door_puller_anchor (Autodesk Fusion 360 design; units mm, degrees)
Autodesk Fusion 360 part; units mm, degrees
note: some values were not read from the file. Set by a fixed rule: which sketch regions a step uses.
sketch "Sketch1" plane through (0, 0, 0) normal (0, 0, 1) x (1, 0, 0)
  line L0 (20, -10) -> (-20, -10)
  line L1 (-20, -10) -> (-20, 10)
  line L2 (-20, 10) -> (20, 10)
  line L3 (20, 10) -> (20, -10)
  line L4 (20, -10) -> (-20, 10) construction
  line L5 (-20, -10) -> (20, 10) construction
  line L6 (10, 10) -> (10, -10)
  line L7 (-10, 10) -> (-10, -10) construction
  circle A0 centre (-10, 0) radius 1.7
  circle A1 centre (-10, 0) radius 3
  circle A2 centre (10, 0) radius 1.45
  circle A3 centre (10, 0) radius 3
  line L8 (-20, 3) -> (20, 3)
  line L9 (-20, -3) -> (20, -3)
  circle A4 centre (10, 0) radius 6
  line L10 (13, 5.1962) -> (13, 10)
  line L11 (7, 5.1962) -> (7, 10)
  line L12 (-7, 3) -> (-7, -3)
  line L13 (7, 3) -> (7, -3)
  line L14 (0, 10) -> (0, -10)
  line L15 (-20, 10) -> (-40, 10)
  line L16 (-40, 10) -> (-40, -10)
  line L17 (-40, -10) -> (-20, -10)
  line L18 (-40, 0) -> (-20, 0) construction
  circle A5 centre (-30, 0) radius 1.7
  circle A6 centre (-30, 0) radius 3
  dimension "d1" = 40
  dimension "d2" = 20
  dimension "d3" = 10
  dimension "d4" = 10
  dimension "d5" = 3.4
  dimension "d6" = 6
  dimension "d7" = 12
  dimension "d8" = 6
  dimension "d15" = 2.9
  dimension "d36" = 20
  constraint horizontal L0
  constraint parallel L0 L2
  constraint parallel L1 L3
  constraint coincident L4 origin
  constraint coincident L5 origin
  constraint coincident L2 L6.start
  constraint coincident L0 L6.end
  constraint vertical L6
  constraint coincident L2 L7.start
  constraint coincident L0 L7.end
  constraint vertical L1
  constraint vertical L7
  constraint midpoint L7 A0.centre
  constraint concentric A0 A1
  constraint coincident L6 A2.centre
  constraint concentric A2 A3
  constraint equal A1 A3
  constraint midpoint L6 A2.centre
  constraint coincident L1 L8.start
  constraint coincident L3 L8.end
  constraint horizontal L8
  constraint tangent A3 L8
  constraint coincident L1 L9.start
  constraint coincident L3 L9.end
  constraint horizontal L9
  constraint tangent A3 L9
  constraint concentric A2 A4
  constraint coincident A4 L10.start
  constraint coincident L2 L10.end
  constraint vertical L10
  constraint symmetric L6 L10.start L11.start
  constraint symmetric L6 L10.end L11.end
  constraint coincident L2 L11.end
  constraint coincident L8 L12.start
  constraint coincident L9 L12.end
  constraint vertical L12
  constraint coincident L8 L13.start
  constraint coincident L9 L13.end
  constraint vertical L13
  constraint tangent A1 L12
  constraint tangent A3 L13
  constraint midpoint L2 L14.start
  constraint coincident L0 L14.end
  constraint vertical L14
  constraint horizontal L15
  constraint vertical L16
  constraint horizontal L17
  constraint midpoint L16 L18.start
  constraint midpoint L1 L18.end
  constraint midpoint L18 A5.centre
  constraint concentric A5 A6
  constraint equal A0 A5
  constraint equal A1 A6
  measures "d1" distance of L1.end L2.end
  measures "d2" distance of L0.end L1.end
  measures "d3" distance of L2.end L6.start
  measures "d4" distance of L1.end L7.start
  measures "d5" diameter of A0
  measures "d6" diameter of A1
  measures "d7" diameter of A4
  measures "d15" diameter of A2
  measures "d36" distance of L1.end L15.end
extrude "Extrude1" add sketch "Sketch1" against normal blind 1.2 contours L8 L9 A4 L14 | L8 L9 L12 L14 | L8 L9 A4 L13
extrude "Extrude2" add sketch "Sketch1" along normal blind 39.5 contours L0 L3 L6 L9 A4 | L0 L6 L9 A4 L14 | L3 L8 L9 A4 | L6 L9 A4 | L6 L9 A4 | L2 L3 L8 A4 L10 | A3 L8 L9 A4 | L8 L9 A4 L14 | L6 A2 A3 | A3 L9 L13 | L6 A2 A3 | L8 L9 A4 L13 | L6 L8 A4 | L2 L8 A4 L11 L14 | L6 A2 | L6 A2 | A3 L8 L13 | L6 L8 A4 | L2 L6 A4 L10 | L2 L6 A4 L11
extrude "Extrude3" cut sketch "Sketch1" along normal blind 39.5 contours L6 A2 | L6 A2
extrude "Extrude4" add sketch "Sketch1" along normal blind 29.5 contours L6 A2 | L6 A2
extrude "Extrude5" add sketch "Sketch1" along normal blind 5 contours L0 L1 L9 L14 | L1 L15 L16 L17 | L8 L9 L12 L14 | L1 A1 L8 L9 | A1 L9 L12 | L1 L2 L8 L14 | A1 | A1 L8 L12 | A6
extrude "Extrude6" add sketch "Sketch1" along normal blind 3 from surface at 5 contours L0 L1 L9 L14 | L1 L15 L16 L17 | L8 L9 L12 L14 | L1 A1 L8 L9 | A1 L9 L12 | L1 L2 L8 L14 | A1 L8 L12
extrude "Extrude8" add sketch "Sketch1" along normal blind 10 from surface at 39.5 contours L0 L3 L6 L9 A4 | L0 L6 L9 A4 L14 | L3 L8 L9 A4 | L2 L3 L8 A4 L10 | L8 L9 A4 L14 | L2 L8 A4 L11 L14
fillet "Fillet3" radius 3 2 edges at (7, 5.1962, 44.5) (13, 5.1962, 44.5)
draft "Draft1" angle 8 neutral plane through (0, 0, 49.5) pull (0, 0, 1) 1 faces at (0, 3.3333, 21.8333)
fillet "Fillet1" radius 3 6 edges at (20, -10, 24.75) (20, 10, 24.75) (-2.9162, 10, 28.75) (-2.9162, -10, 28.75) (-40, -10, 4) (-40, 10, 4)
chamfer "Chamfer1" distance 0.4 angle 45 2 edges at (-12.797, 1.0848, 8) (-32.797, 1.0848, 8)
chamfer "Chamfer2" distance 0.2 angle 45 2 edges at (-11.585, 0.6147, 5) (-31.585, 0.6147, 5)
chamfer "Chamfer3" distance 0.2 angle 45 1 edges at (8.6481, 0.5243, 39.5)
chamfer "Chamfer4" distance 1 angle 45 5 edges at (-19.9015, 10, 8) (-39.1213, 9.1213, 8) (-40, 0, 8) (-39.1213, -9.1213, 8) (-19.9015, -10, 8)
extrude "Extrude7" cut 1 faces at (-2.3333, 1, -1.2) along direction (0, 0, 1) blind 1.2
chamfer "Chamfer5" distance 0.4 angle 45 1 faces at (8.5667, 0, 0)
fillet "Fillet4" radius 1.5 2 edges at (7, 10, 44.5) (13, 10, 44.5)
chamfer "Chamfer6" distance 1 angle 45 16 edges at (0, 0, 49.5) (0.8873, -9.1213, 49.5) (10.0147, -10, 49.5) (19.1213, -9.1213, 49.5) (20, 0, 49.5) (19.1213, 9.1213, 49.5) (15.75, 10, 49.5) (13.4393, 9.5607, 49.5) (13, 7.6041, 49.5) (13.2614, 5.4835, 49.5) (10, -6, 49.5) (6.7386, 5.4835, 49.5) (7, 7.6041, 49.5) (6.5607, 9.5607, 49.5) (4.2647, 10, 49.5) (0.8873, 9.1213, 49.5)
equation "d9 = -( 2 mm - 0.8 mm )"
equation "d16 = 39.50 mm - 10 mm"
